Autodesk Fusion 360 part; units mm, degrees
(part 8 of 9)
  spline S13 degree 5 poles (-16.6117, 12.3429) (-16.6198, 12.3478) (-16.6358, 12.3576) (-16.6595, 12.373) (-16.6903, 12.3947) (-16.7276, 12.4235) (-16.7642, 12.4534) (-16.8004, 12.484) (-16.8362, 12.5151) (-16.8719, 12.5464) (-16.9074, 12.578) (-16.9427, 12.61) (-16.9776, 12.6425) (-17.0121, 12.6755) (-17.0463, 12.709) (-17.0801, 12.7431) (-17.1135, 12.7776) (-17.1467, 12.8125) (-17.1796, 12.8477) (-17.2124, 12.8832) (-17.2449, 12.919) (-17.2771, 12.9552) (-17.3091, 12.9916) (-17.3409, 13.0284) (-17.3723, 13.0655) (-17.4036, 13.103) (-17.4346, 13.1407) (-17.4653, 13.1788) (-17.4959, 13.2171) (-17.5262, 13.2557) (-17.5563, 13.2945) (-17.5862, 13.3337) (-17.6158, 13.373) (-17.6453, 13.4127) (-17.6745, 13.4526) (-17.7035, 13.4928) (-17.7323, 13.5332) (-17.7609, 13.5738) (-17.7892, 13.6147) (-17.8174, 13.6559) (-17.8454, 13.6972) (-17.8731, 13.7388) (-17.9007, 13.7807) (-17.928, 13.8227) (-17.9551, 13.865) (-17.9821, 13.9075) (-18.0088, 13.9502) (-18.0354, 13.9931) (-18.0617, 14.0363) (-18.0878, 14.0796) (-18.1138, 14.1232) (-18.1395, 14.1669) (-18.165, 14.2109) (-18.1904, 14.255) (-18.2156, 14.2994) (-18.2405, 14.344) (-18.2653, 14.3887) (-18.2898, 14.4336) (-18.3142, 14.4788) (-18.3384, 14.5241) (-18.3624, 14.5696) (-18.3862, 14.6153) (-18.4098, 14.6612) (-18.4332, 14.7072) (-18.4564, 14.7535) (-18.4795, 14.7999) (-18.5023, 14.8465) (-18.525, 14.8932) (-18.5474, 14.9401) (-18.5697, 14.9873) (-18.5918, 15.0345) (-18.6093, 15.0725) (-18.6224, 15.101) (-18.631, 15.1201) (-18.6354, 15.1296) knots 0 0 0 0 0 0 0.01428571 0.02857143 0.04285714 0.05714286 0.07142857 0.08571429 0.1 0.11428571 0.12857143 0.14285714 0.15714286 0.17142857 0.18571429 0.2 0.21428571 0.22857143 0.24285714 0.25714286 0.27142857 0.28571429 0.3 0.31428571 0.32857143 0.34285714 0.35714286 0.37142857 0.38571429 0.4 0.41428571 0.42857143 0.44285714 0.45714286 0.47142857 0.48571429 0.5 0.51428571 0.52857143 0.54285714 0.55714286 0.57142857 0.58571429 0.6 0.61428571 0.62857143 0.64285714 0.65714286 0.67142857 0.68571429 0.7 0.71428571 0.72857143 0.74285714 0.75714286 0.77142857 0.78571429 0.8 0.81428571 0.82857143 0.84285714 0.85714286 0.87142857 0.88571429 0.9 0.91428571 0.92857143 0.94285714 0.95714286 0.97142857 0.98571429 1 1 1 1 1 1
  line L13 (-16.6117, 12.3429) -> (-16.2962, 12.1549)
  arc A27 (-15.962, 10.9599) -> (-16.2962, 12.1549) centre (-16.757, 11.3818) ccw
  arc A28 (-15.962, 10.9599) -> (-16.228, 10.4378) centre (-0.4607, 2.7328) ccw
  arc A29 (-17.3912, 10.0058) -> (-16.228, 10.4378) centre (-17.0366, 10.833) ccw
  line L14 (-17.3912, 10.0058) -> (-17.7288, 10.1505)
  spline S14 degree 5 poles (-17.7288, 10.1505) (-17.7375, 10.1542) (-17.7549, 10.1614) (-17.7812, 10.1715) (-17.8169, 10.1836) (-17.8621, 10.197) (-17.9078, 10.209) (-17.9538, 10.2202) (-18.0001, 10.231) (-18.0464, 10.2414) (-18.0928, 10.2516) (-18.1394, 10.2613) (-18.1862, 10.2705) (-18.2332, 10.279) (-18.2804, 10.2869) (-18.3278, 10.2942) (-18.3754, 10.301) (-18.4232, 10.3073) (-18.471, 10.3133) (-18.519, 10.3189) (-18.567, 10.3241) (-18.6152, 10.329) (-18.6635, 10.3334) (-18.7119, 10.3375) (-18.7605, 10.3411) (-18.8091, 10.3444) (-18.8579, 10.3473) (-18.9068, 10.3498) (-18.9557, 10.352) (-19.0047, 10.3538) (-19.0539, 10.3553) (-19.1031, 10.3565) (-19.1524, 10.3574) (-19.2018, 10.3579) (-19.2512, 10.3581) (-19.3008, 10.3579) (-19.3504, 10.3575) (-19.4001, 10.3567) (-19.4499, 10.3556) (-19.4997, 10.3542) (-19.5496, 10.3525) (-19.5996, 10.3505) (-19.6496, 10.3482) (-19.6997, 10.3456) (-19.7498, 10.3427) (-19.8, 10.3395) (-19.8503, 10.3361) (-19.9006, 10.3323) (-19.951, 10.3282) (-20.0014, 10.3239) (-20.0519, 10.3193) (-20.1025, 10.3144) (-20.153, 10.3092) (-20.2037, 10.3038) (-20.2543, 10.2981) (-20.3051, 10.2921) (-20.3558, 10.2858) (-20.4066, 10.2793) (-20.4574, 10.2724) (-20.5083, 10.2654) (-20.5592, 10.258) (-20.6102, 10.2504) (-20.6612, 10.2426) (-20.7122, 10.2344) (-20.7633, 10.2261) (-20.8144, 10.2174) (-20.8655, 10.2085) (-20.9166, 10.1994) (-20.9678, 10.1899) (-21.019, 10.1803) (-21.0702, 10.1704) (-21.1112, 10.1622) (-21.142, 10.156) (-21.1625, 10.1518) (-21.1728, 10.1497) knots 0 0 0 0 0 0 0.01428571 0.02857143 0.04285714 0.05714286 0.07142857 0.08571429 0.1 0.11428571 0.12857143 0.14285714 0.15714286 0.17142857 0.18571429 0.2 0.21428571 0.22857143 0.24285714 0.25714286 0.27142857 0.28571429 0.3 0.31428571 0.32857143 0.34285714 0.35714286 0.37142857 0.38571429 0.4 0.41428571 0.42857143 0.44285714 0.45714286 0.47142857 0.48571429 0.5 0.51428571 0.52857143 0.54285714 0.55714286 0.57142857 0.58571429 0.6 0.61428571 0.62857143 0.64285714 0.65714286 0.67142857 0.68571429 0.7 0.71428571 0.72857143 0.74285714 0.75714286 0.77142857 0.78571429 0.8 0.81428571 0.82857143 0.84285714 0.85714286 0.87142857 0.88571429 0.9 0.91428571 0.92857143 0.94285714 0.95714286 0.97142857 0.98571429 1 1 1 1 1 1
  arc A30 (-21.1728, 10.1497) -> (-21.5767, 8.9066) centre (-0.4607, 2.7328) ccw
  spline S15 degree 5 poles (-18.7909, 6.8816) (-18.8001, 6.8837) (-18.8184, 6.8881) (-18.8457, 6.8955) (-18.8816, 6.9066) (-18.9261, 6.9224) (-18.9701, 6.9396) (-19.0139, 6.9575) (-19.0577, 6.976) (-19.1013, 6.9948) (-19.1448, 7.0138) (-19.1882, 7.0334) (-19.2315, 7.0534) (-19.2745, 7.0742) (-19.3174, 7.0955) (-19.36, 7.1175) (-19.4025, 7.14) (-19.4448, 7.1629) (-19.487, 7.1862) (-19.5291, 7.2099) (-19.5711, 7.2339) (-19.6129, 7.2583) (-19.6546, 7.2831) (-19.6962, 7.3082) (-19.7376, 7.3338) (-19.7789, 7.3598) (-19.82, 7.3861) (-19.861, 7.4128) (-19.9019, 7.4398) (-19.9427, 7.4671) (-19.9833, 7.4948) (-20.0238, 7.5228) (-20.0642, 7.551) (-20.1045, 7.5797) (-20.1446, 7.6086) (-20.1846, 7.6378) (-20.2245, 7.6674) (-20.2642, 7.6972) (-20.3038, 7.7273) (-20.3433, 7.7577) (-20.3827, 7.7884) (-20.422, 7.8194) (-20.4611, 7.8507) (-20.5001, 7.8822) (-20.5389, 7.9141) (-20.5777, 7.9462) (-20.6163, 7.9785) (-20.6548, 8.0111) (-20.6932, 8.044) (-20.7315, 8.0772) (-20.7696, 8.1106) (-20.8076, 8.1442) (-20.8455, 8.1782) (-20.8832, 8.2123) (-20.9208, 8.2467) (-20.9584, 8.2814) (-20.9957, 8.3163) (-21.033, 8.3515) (-21.0701, 8.3868) (-21.1071, 8.4225) (-21.144, 8.4583) (-21.1808, 8.4944) (-21.2174, 8.5308) (-21.2539, 8.5673) (-21.2903, 8.6041) (-21.3265, 8.6412) (-21.3626, 8.6784) (-21.3986, 8.7159) (-21.4345, 8.7536) (-21.4702, 8.7915) (-21.5059, 8.8296) (-21.5342, 8.8603) (-21.5555, 8.8834) (-21.5696, 8.8989) (-21.5767, 8.9066) knots 0 0 0 0 0 0 0.01428571 0.02857143 0.04285714 0.05714286 0.07142857 0.08571429 0.1 0.11428571 0.12857143 0.14285714 0.15714286 0.17142857 0.18571429 0.2 0.21428571 0.22857143 0.24285714 0.25714286 0.27142857 0.28571429 0.3 0.31428571 0.32857143 0.34285714 0.35714286 0.37142857 0.38571429 0.4 0.41428571 0.42857143 0.44285714 0.45714286 0.47142857 0.48571429 0.5 0.51428571 0.52857143 0.54285714 0.55714286 0.57142857 0.58571429 0.6 0.61428571 0.62857143 0.64285714 0.65714286 0.67142857 0.68571429 0.7 0.71428571 0.72857143 0.74285714 0.75714286 0.77142857 0.78571429 0.8 0.81428571 0.82857143 0.84285714 0.85714286 0.87142857 0.88571429 0.9 0.91428571 0.92857143 0.94285714 0.95714286 0.97142857 0.98571429 1 1 1 1 1 1
  line L15 (-18.7909, 6.8816) -> (-18.4327, 6.8003)
  arc A31 (-17.7456, 5.767) -> (-18.4327, 6.8003) centre (-18.6321, 5.9227) ccw
  arc A32 (-17.7456, 5.767) -> (-17.8373, 5.1884) centre (-0.4607, 2.7328) ccw
  arc A33 (-18.8101, 4.418) -> (-17.8373, 5.1884) centre (-18.7284, 5.3143) ccw
  line L16 (-18.8101, 4.418) -> (-19.1758, 4.4513)
  spline S16 degree 5 poles (-19.1758, 4.4513) (-19.1852, 4.4522) (-19.204, 4.4536) (-19.2322, 4.4551) (-19.2698, 4.4556) (-19.317, 4.4543) (-19.3642, 4.4516) (-19.4114, 4.4481) (-19.4587, 4.444) (-19.506, 4.4396) (-19.5533, 4.4349) (-19.6006, 4.4298) (-19.6479, 4.4241) (-19.6953, 4.4177) (-19.7426, 4.4106) (-19.79, 4.4029) (-19.8373, 4.3946) (-19.8847, 4.3859) (-19.932, 4.3768) (-19.9794, 4.3673) (-20.0267, 4.3574) (-20.074, 4.3471) (-20.1213, 4.3365) (-20.1686, 4.3253) (-20.2159, 4.3138) (-20.2632, 4.3019) (-20.3105, 4.2895) (-20.3577, 4.2769) (-20.405, 4.2638) (-20.4522, 4.2504) (-20.4994, 4.2367) (-20.5465, 4.2226) (-20.5937, 4.2082) (-20.6408, 4.1934) (-20.6879, 4.1783) (-20.735, 4.1628) (-20.782, 4.1471) (-20.829, 4.131) (-20.876, 4.1145) (-20.923, 4.0978) (-20.9699, 4.0808) (-21.0168, 4.0634) (-21.0637, 4.0458) (-21.1105, 4.0279) (-21.1574, 4.0096) (-21.2041, 3.9911) (-21.2509, 3.9722) (-21.2976, 3.9531) (-21.3442, 3.9337) (-21.3908, 3.914) (-21.4374, 3.894) (-21.484, 3.8737) (-21.5305, 3.8532) (-21.5769, 3.8323) (-21.6234, 3.8112) (-21.6697, 3.7898) (-21.7161, 3.7682) (-21.7624, 3.7463) (-21.8086, 3.7241) (-21.8548, 3.7016) (-21.901, 3.6789) (-21.9471, 3.656) (-21.9932, 3.6327) (-22.0392, 3.6092) (-22.0851, 3.5855) (-22.1311, 3.5615) (-22.1769, 3.5372) (-22.2227, 3.5127) (-22.2685, 3.4879) (-22.3142, 3.4629) (-22.3599, 3.4376) (-22.3963, 3.4172) (-22.4237, 3.4018) (-22.4419, 3.3915) (-22.451, 3.3863) knots 0 0 0 0 0 0 0.01428571 0.02857143 0.04285714 0.05714286 0.07142857 0.08571429 0.1 0.11428571 0.12857143 0.14285714 0.15714286 0.17142857 0.18571429 0.2 0.21428571 0.22857143 0.24285714 0.25714286 0.27142857 0.28571429 0.3 0.31428571 0.32857143 0.34285714 0.35714286 0.37142857 0.38571429 0.4 0.41428571 0.42857143 0.44285714 0.45714286 0.47142857 0.48571429 0.5 0.51428571 0.52857143 0.54285714 0.55714286 0.57142857 0.58571429 0.6 0.61428571 0.62857143 0.64285714 0.65714286 0.67142857 0.68571429 0.7 0.71428571 0.72857143 0.74285714 0.75714286 0.77142857 0.78571429 0.8 0.81428571 0.82857143 0.84285714 0.85714286 0.87142857 0.88571429 0.9 0.91428571 0.92857143 0.94285714 0.95714286 0.97142857 0.98571429 1 1 1 1 1 1
  arc A34 (-22.451, 3.3863) -> (-22.451, 2.0792) centre (-0.4607, 2.7328) ccw
  spline S17 degree 5 poles (-19.1758, 1.0142) (-19.1852, 1.0134) (-19.204, 1.0119) (-19.2322, 1.0105) (-19.2698, 1.01) (-19.317, 1.0112) (-19.3642, 1.0139) (-19.4114, 1.0175) (-19.4587, 1.0215) (-19.506, 1.0259) (-19.5533, 1.0306) (-19.6006, 1.0358) (-19.6479, 1.0415) (-19.6953, 1.0479) (-19.7426, 1.055) (-19.79, 1.0627) (-19.8373, 1.071) (-19.8847, 1.0797) (-19.932, 1.0888) (-19.9794, 1.0983) (-20.0267, 1.1082) (-20.074, 1.1184) (-20.1213, 1.1291) (-20.1686, 1.1402) (-20.2159, 1.1517) (-20.2632, 1.1637) (-20.3105, 1.176) (-20.3577, 1.1887) (-20.405, 1.2018) (-20.4522, 1.2152) (-20.4994, 1.2289) (-20.5465, 1.243) (-20.5937, 1.2574) (-20.6408, 1.2722) (-20.6879, 1.2873) (-20.735, 1.3027) (-20.782, 1.3185) (-20.829, 1.3346) (-20.876, 1.351) (-20.923, 1.3677) (-20.9699, 1.3848) (-21.0168, 1.4021) (-21.0637, 1.4198) (-21.1105, 1.4377) (-21.1574, 1.456) (-21.2041, 1.4745) (-21.2509, 1.4933) (-21.2976, 1.5125) (-21.3442, 1.5319) (-21.3908, 1.5516) (-21.4374, 1.5716) (-21.484, 1.5919) (-21.5305, 1.6124) (-21.5769, 1.6332) (-21.6234, 1.6543) (-21.6697, 1.6757) (-21.7161, 1.6974) (-21.7624, 1.7193) (-21.8086, 1.7415) (-21.8548, 1.7639) (-21.901, 1.7866) (-21.9471, 1.8096) (-21.9932, 1.8328) (-22.0392, 1.8563) (-22.0851, 1.8801) (-22.1311, 1.9041) (-22.1769, 1.9284) (-22.2227, 1.9529) (-22.2685, 1.9776) (-22.3142, 2.0026) (-22.3599, 2.0279) (-22.3963, 2.0483) (-22.4237, 2.0637) (-22.4419, 2.0741) (-22.451, 2.0792) knots 0 0 0 0 0 0 0.01428571 0.02857143 0.04285714 0.05714286 0.07142857 0.08571429 0.1 0.11428571 0.12857143 0.14285714 0.15714286 0.17142857 0.18571429 0.2 0.21428571 0.22857143 0.24285714 0.25714286 0.27142857 0.28571429 0.3 0.31428571 0.32857143 0.34285714 0.35714286 0.37142857 0.38571429 0.4 0.41428571 0.42857143 0.44285714 0.45714286 0.47142857 0.48571429 0.5 0.51428571 0.52857143 0.54285714 0.55714286 0.57142857 0.58571429 0.6 0.61428571 0.62857143 0.64285714 0.65714286 0.67142857 0.68571429 0.7 0.71428571 0.72857143 0.74285714 0.75714286 0.77142857 0.78571429 0.8 0.81428571 0.82857143 0.84285714 0.85714286 0.87142857 0.88571429 0.9 0.91428571 0.92857143 0.94285714 0.95714286 0.97142857 0.98571429 1 1 1 1 1 1
  line L17 (-19.1758, 1.0142) -> (-18.8101, 1.0476)
  arc A35 (-17.8373, 0.2772) -> (-18.8101, 1.0476) centre (-18.7284, 0.1513) ccw
  arc A36 (-17.8373, 0.2772) -> (-17.7456, -0.3015) centre (-0.4607, 2.7328) ccw
  arc A37 (-18.4327, -1.3347) -> (-17.7456, -0.3015) centre (-18.6321, -0.4571) ccw
  line L18 (-18.4327, -1.3347) -> (-18.7909, -1.4161)
  spline S18 degree 5 poles (-18.7909, -1.4161) (-18.8001, -1.4182) (-18.8184, -1.4226) (-18.8457, -1.4299) (-18.8816, -1.4411) (-18.9261, -1.4569) (-18.9701, -1.474) (-19.0139, -1.492) (-19.0577, -1.5104) (-19.1013, -1.5292) (-19.1448, -1.5483) (-19.1882, -1.5678) (-19.2315, -1.5879) (-19.2745, -1.6086) (-19.3174, -1.63) (-19.36, -1.6519) (-19.4025, -1.6744) (-19.4448, -1.6974) (-19.487, -1.7207) (-19.5291, -1.7443) (-19.5711, -1.7683) (-19.6129, -1.7927) (-19.6546, -1.8175) (-19.6962, -1.8427) (-19.7376, -1.8683) (-19.7789, -1.8942) (-19.82, -1.9206) (-19.861, -1.9472) (-19.9019, -1.9742) (-19.9427, -2.0016) (-19.9833, -2.0292) (-20.0238, -2.0572) (-20.0642, -2.0855) (-20.1045, -2.1141) (-20.1446, -2.143) (-20.1846, -2.1723) (-20.2245, -2.2018) (-20.2642, -2.2316) (-20.3038, -2.2618) (-20.3433, -2.2922) (-20.3827, -2.3229) (-20.422, -2.3539) (-20.4611, -2.3851) (-20.5001, -2.4167) (-20.5389, -2.4485) (-20.5777, -2.4806) (-20.6163, -2.513) (-20.6548, -2.5456) (-20.6932, -2.5785) (-20.7315, -2.6116) (-20.7696, -2.645) (-20.8076, -2.6787) (-20.8455, -2.7126) (-20.8832, -2.7468) (-20.9208, -2.7812) (-20.9584, -2.8158) (-20.9957, -2.8507) (-21.033, -2.8859) (-21.0701, -2.9213) (-21.1071, -2.9569) (-21.144, -2.9928) (-21.1808, -3.0289) (-21.2174, -3.0652) (-21.2539, -3.1018) (-21.2903, -3.1386) (-21.3265, -3.1756) (-21.3626, -3.2128) (-21.3986, -3.2503) (-21.4345, -3.288) (-21.4702, -3.3259) (-21.5059, -3.3641) (-21.5342, -3.3947) (-21.5555, -3.4179) (-21.5696, -3.4333) (-21.5767, -3.441) knots 0 0 0 0 0 0 0.01428571 0.02857143 0.04285714 0.05714286 0.07142857 0.08571429 0.1 0.11428571 0.12857143 0.14285714 0.15714286 0.17142857 0.18571429 0.2 0.21428571 0.22857143 0.24285714 0.25714286 0.27142857 0.28571429 0.3 0.31428571 0.32857143 0.34285714 0.35714286 0.37142857 0.38571429 0.4 0.41428571 0.42857143 0.44285714 0.45714286 0.47142857 0.48571429 0.5 0.51428571 0.52857143 0.54285714 0.55714286 0.57142857 0.58571429 0.6 0.61428571 0.62857143 0.64285714 0.65714286 0.67142857 0.68571429 0.7 0.71428571 0.72857143 0.74285714 0.75714286 0.77142857 0.78571429 0.8 0.81428571 0.82857143 0.84285714 0.85714286 0.87142857 0.88571429 0.9 0.91428571 0.92857143 0.94285714 0.95714286 0.97142857 0.98571429 1 1 1 1 1 1
  arc A38 (-21.5767, -3.441) -> (-21.1728, -4.6841) centre (-0.4607, 2.7328) ccw
  spline S19 degree 5 poles (-17.7288, -4.6849) (-17.7375, -4.6886) (-17.7549, -4.6958) (-17.7812, -4.7059) (-17.8169, -4.7181) (-17.8621, -4.7314) (-17.9078, -4.7434) (-17.9538, -4.7546) (-18.0001, -4.7654) (-18.0464, -4.7759) (-18.0928, -4.786) (-18.1394, -4.7957) (-18.1862, -4.8049) (-18.2332, -4.8135) (-18.2804, -4.8213) (-18.3278, -4.8286) (-18.3754, -4.8354) (-18.4232, -4.8417) (-18.471, -4.8477) (-18.519, -4.8533) (-18.567, -4.8585) (-18.6152, -4.8634) (-18.6635, -4.8679) (-18.7119, -4.8719) (-18.7605, -4.8756) (-18.8091, -4.8788) (-18.8579, -4.8817) (-18.9068, -4.8842) (-18.9557, -4.8864) (-19.0047, -4.8883) (-19.0539, -4.8898) (-19.1031, -4.891) (-19.1524, -4.8918) (-19.2018, -4.8923) (-19.2512, -4.8925) (-19.3008, -4.8924) (-19.3504, -4.8919) (-19.4001, -4.8911) (-19.4499, -4.89) (-19.4997, -4.8886) (-19.5496, -4.887) (-19.5996, -4.885) (-19.6496, -4.8827) (-19.6997, -4.8801) (-19.7498, -4.8772) (-19.8, -4.874) (-19.8503, -4.8705) (-19.9006, -4.8667) (-19.951, -4.8627) (-20.0014, -4.8584) (-20.0519, -4.8537) (-20.1025, -4.8488) (-20.153, -4.8437) (-20.2037, -4.8382) (-20.2543, -4.8325) (-20.3051, -4.8265) (-20.3558, -4.8202) (-20.4066, -4.8137) (-20.4574, -4.8069) (-20.5083, -4.7998) (-20.5592, -4.7925) (-20.6102, -4.7849) (-20.6612, -4.777) (-20.7122, -4.7689) (-20.7633, -4.7605) (-20.8144, -4.7519) (-20.8655, -4.743) (-20.9166, -4.7338) (-20.9678, -4.7244) (-21.019, -4.7147) (-21.0702, -4.7048) (-21.1112, -4.6967) (-21.142, -4.6904) (-21.1625, -4.6863) (-21.1728, -4.6841) knots 0 0 0 0 0 0 0.01428571 0.02857143 0.04285714 0.05714286 0.07142857 0.08571429 0.1 0.11428571 0.12857143 0.14285714 0.15714286 0.17142857 0.18571429 0.2 0.21428571 0.22857143 0.24285714 0.25714286 0.27142857 0.28571429 0.3 0.31428571 0.32857143 0.34285714 0.35714286 0.37142857 0.38571429 0.4 0.41428571 0.42857143 0.44285714 0.45714286 0.47142857 0.48571429 0.5 0.51428571 0.52857143 0.54285714 0.55714286 0.57142857 0.58571429 0.6 0.61428571 0.62857143 0.64285714 0.65714286 0.67142857 0.68571429 0.7 0.71428571 0.72857143 0.74285714 0.75714286 0.77142857 0.78571429 0.8 0.81428571 0.82857143 0.84285714 0.85714286 0.87142857 0.88571429 0.9 0.91428571 0.92857143 0.94285714 0.95714286 0.97142857 0.98571429 1 1 1 1 1 1
  line L19 (-17.7288, -4.6849) -> (-17.3912, -4.5402)
  arc A39 (-16.228, -4.9723) -> (-17.3912, -4.5402) centre (-17.0366, -5.3674) ccw
  arc A40 (-16.228, -4.9723) -> (-15.962, -5.4943) centre (-0.4607, 2.7328) ccw
  arc A41 (-16.2962, -6.6893) -> (-15.962, -5.4943) centre (-16.757, -5.9162) ccw
  line L20 (-16.2962, -6.6893) -> (-16.6117, -6.8774)
  spline S20 degree 5 poles (-16.6117, -6.8774) (-16.6198, -6.8822) (-16.6358, -6.892) (-16.6595, -6.9074) (-16.6903, -6.9292) (-16.7276, -6.9579) (-16.7642, -6.9878) (-16.8004, -7.0185) (-16.8362, -7.0495) (-16.8719, -7.0809) (-16.9074, -7.1125) (-16.9427, -7.1444) (-16.9776, -7.1769) (-17.0121, -7.2099) (-17.0463, -7.2435) (-17.0801, -7.2775) (-17.1135, -7.3121) (-17.1467, -7.3469) (-17.1796, -7.3822) (-17.2124, -7.4177) (-17.2449, -7.4535) (-17.2771, -7.4896) (-17.3091, -7.526) (-17.3409, -7.5628) (-17.3723, -7.6) (-17.4036, -7.6374) (-17.4346, -7.6752) (-17.4653, -7.7132) (-17.4959, -7.7515) (-17.5262, -7.7901) (-17.5563, -7.829) (-17.5862, -7.8681) (-17.6158, -7.9075) (-17.6453, -7.9471) (-17.6745, -7.987) (-17.7035, -8.0272) (-17.7323, -8.0676) (-17.7609, -8.1083) (-17.7892, -8.1492) (-17.8174, -8.1903) (-17.8454, -8.2317) (-17.8731, -8.2733) (-17.9007, -8.3151) (-17.928, -8.3572) (-17.9551, -8.3994) (-17.9821, -8.4419) (-18.0088, -8.4846) (-18.0354, -8.5276) (-18.0617, -8.5707) (-18.0878, -8.614) (-18.1138, -8.6576) (-18.1395, -8.7014) (-18.165, -8.7453) (-18.1904, -8.7895) (-18.2156, -8.8338) (-18.2405, -8.8784) (-18.2653, -8.9231) (-18.2898, -8.9681) (-18.3142, -9.0132) (-18.3384, -9.0585) (-18.3624, -9.104) (-18.3862, -9.1497) (-18.4098, -9.1956) (-18.4332, -9.2417) (-18.4564, -9.2879) (-18.4795, -9.3343) (-18.5023, -9.3809) (-18.525, -9.4277) (-18.5474, -9.4746) (-18.5697, -9.5217) (-18.5918, -9.569) (-18.6093, -9.6069) (-18.6224, -9.6355) (-18.631, -9.6545) (-18.6354, -9.6641) knots 0 0 0 0 0 0 0.01428571 0.02857143 0.04285714 0.05714286 0.07142857 0.08571429 0.1 0.11428571 0.12857143 0.14285714 0.15714286 0.17142857 0.18571429 0.2 0.21428571 0.22857143 0.24285714 0.25714286 0.27142857 0.28571429 0.3 0.31428571 0.32857143 0.34285714 0.35714286 0.37142857 0.38571429 0.4 0.41428571 0.42857143 0.44285714 0.45714286 0.47142857 0.48571429 0.5 0.51428571 0.52857143 0.54285714 0.55714286 0.57142857 0.58571429 0.6 0.61428571 0.62857143 0.64285714 0.65714286 0.67142857 0.68571429 0.7 0.71428571 0.72857143 0.74285714 0.75714286 0.77142857 0.78571429 0.8 0.81428571 0.82857143 0.84285714 0.85714286 0.87142857 0.88571429 0.9 0.91428571 0.92857143 0.94285714 0.95714286 0.97142857 0.98571429 1 1 1 1 1 1
  arc A42 (-18.6354, -9.6641) -> (-17.8671, -10.7215) centre (-0.4607, 2.7328) ccw
  spline S21 degree 5 poles (-14.5914, -9.658) (-14.5985, -9.6642) (-14.6129, -9.6764) (-14.6348, -9.6942) (-14.665, -9.7167) (-14.7039, -9.7434) (-14.7436, -9.769) (-14.7839, -9.7938) (-14.8246, -9.8184) (-14.8654, -9.8426) (-14.9064, -9.8666) (-14.9477, -9.8903) (-14.9894, -9.9135) (-15.0314, -9.9361) (-15.0739, -9.9582) (-15.1168, -9.9798) (-15.1599, -10.0009) (-15.2034, -10.0217) (-15.247, -10.0422) (-15.2909, -10.0623) (-15.335, -10.0822) (-15.3793, -10.1017) (-15.4239, -10.1208) (-15.4687, -10.1397) (-15.5137, -10.1581) (-15.559, -10.1763) (-15.6045, -10.1941) (-15.6502, -10.2116) (-15.696, -10.2288) (-15.7421, -10.2457) (-15.7884, -10.2623) (-15.8348, -10.2786) (-15.8814, -10.2947) (-15.9282, -10.3104) (-15.9752, -10.3259) (-16.0224, -10.3411) (-16.0697, -10.356) (-16.1172, -10.3706) (-16.1649, -10.3849) (-16.2127, -10.399) (-16.2607, -10.4128) (-16.3088, -10.4263) (-16.3571, -10.4396) (-16.4056, -10.4526) (-16.4541, -10.4654) (-16.5029, -10.4779) (-16.5518, -10.4901) (-16.6008, -10.5021) (-16.65, -10.5138) (-16.6993, -10.5252) (-16.7487, -10.5364) (-16.7983, -10.5474) (-16.848, -10.5581) (-16.8978, -10.5686) (-16.9478, -10.5788) (-16.9979, -10.5888) (-17.0481, -10.5985) (-17.0984, -10.608) (-17.1489, -10.6172) (-17.1994, -10.6262) (-17.2501, -10.635) (-17.3009, -10.6435) (-17.3519, -10.6517) (-17.4029, -10.6598) (-17.454, -10.6676) (-17.5053, -10.6752) (-17.5567, -10.6825) (-17.6081, -10.6896) (-17.6597, -10.6964) (-17.7114, -10.7031) (-17.7632, -10.7095) (-17.8047, -10.7144) (-17.8359, -10.718) (-17.8567, -10.7203) (-17.8671, -10.7215) knots 0 0 0 0 0 0 0.01428571 0.02857143 0.04285714 0.05714286 0.07142857 0.08571429 0.1 0.11428571 0.12857143 0.14285714 0.15714286 0.17142857 0.18571429 0.2 0.21428571 0.22857143 0.24285714 0.25714286 0.27142857 0.28571429 0.3 0.31428571 0.32857143 0.34285714 0.35714286 0.37142857 0.38571429 0.4 0.41428571 0.42857143 0.44285714 0.45714286 0.47142857 0.48571429 0.5 0.51428571 0.52857143 0.54285714 0.55714286 0.57142857 0.58571429 0.6 0.61428571 0.62857143 0.64285714 0.65714286 0.67142857 0.68571429 0.7 0.71428571 0.72857143 0.74285714 0.75714286 0.77142857 0.78571429 0.8 0.81428571 0.82857143 0.84285714 0.85714286 0.87142857 0.88571429 0.9 0.91428571 0.92857143 0.94285714 0.95714286 0.97142857 0.98571429 1 1 1 1 1 1
  line L21 (-14.5914, -9.658) -> (-14.3151, -9.4161)
  arc A43 (-13.0753, -9.4675) -> (-14.3151, -9.4161) centre (-13.7222, -10.0932) ccw
  arc A44 (-13.0753, -9.4675) -> (-12.661, -9.8818) centre (-0.4607, 2.7328) ccw
  arc A45 (-12.6096, -11.1216) -> (-12.661, -9.8818) centre (-13.2867, -10.5287) ccw
  line L22 (-12.6096, -11.1216) -> (-12.8515, -11.3979)
  spline S22 degree 5 poles (-12.8515, -11.3979) (-12.8577, -11.405) (-12.8699, -11.4194) (-12.8877, -11.4413) (-12.9102, -11.4715) (-12.9369, -11.5104) (-12.9625, -11.5501) (-12.9873, -11.5904) (-13.0119, -11.6311) (-13.0361, -11.6719) (-13.0601, -11.7129) (-13.0838, -11.7542) (-13.107, -11.7959) (-13.1296, -11.8379) (-13.1517, -11.8804) (-13.1733, -11.9233) (-13.1944, -11.9664) (-13.2152, -12.0099) (-13.2357, -12.0535) (-13.2558, -12.0974) (-13.2757, -12.1415) (-13.2952, -12.1858) (-13.3143, -12.2304) (-13.3332, -12.2752) (-13.3516, -12.3202) (-13.3698, -12.3655) (-13.3876, -12.411) (-13.4051, -12.4567) (-13.4223, -12.5025) (-13.4392, -12.5486) (-13.4558, -12.5949) (-13.4721, -12.6413) (-13.4882, -12.6879) (-13.5039, -12.7347) (-13.5194, -12.7817) (-13.5346, -12.8289) (-13.5495, -12.8762) (-13.5641, -12.9237) (-13.5784, -12.9714) (-13.5925, -13.0192) (-13.6063, -13.0672) (-13.6198, -13.1153) (-13.6331, -13.1636) (-13.6461, -13.2121) (-13.6589, -13.2607) (-13.6714, -13.3094) (-13.6836, -13.3583) (-13.6956, -13.4073) (-13.7073, -13.4565) (-13.7187, -13.5058) (-13.7299, -13.5552) (-13.7409, -13.6048) (-13.7516, -13.6545) (-13.7621, -13.7043) (-13.7723, -13.7543) (-13.7823, -13.8044) (-13.792, -13.8546) (-13.8015, -13.9049) (-13.8107, -13.9554) (-13.8197, -14.0059) (-13.8284, -14.0566) (-13.837, -14.1074) (-13.8452, -14.1584) (-13.8533, -14.2094) (-13.8611, -14.2605) (-13.8686, -14.3118) (-13.876, -14.3632) (-13.8831, -14.4146) (-13.8899, -14.4662) (-13.8966, -14.5179) (-13.903, -14.5697) (-13.9079, -14.6112) (-13.9115, -14.6424) (-13.9138, -14.6632) (-13.915, -14.6736) knots 0 0 0 0 0 0 0.01428571 0.02857143 0.04285714 0.05714286 0.07142857 0.08571429 0.1 0.11428571 0.12857143 0.14285714 0.15714286 0.17142857 0.18571429 0.2 0.21428571 0.22857143 0.24285714 0.25714286 0.27142857 0.28571429 0.3 0.31428571 0.32857143 0.34285714 0.35714286 0.37142857 0.38571429 0.4 0.41428571 0.42857143 0.44285714 0.45714286 0.47142857 0.48571429 0.5 0.51428571 0.52857143 0.54285714 0.55714286 0.57142857 0.58571429 0.6 0.61428571 0.62857143 0.64285714 0.65714286 0.67142857 0.68571429 0.7 0.71428571 0.72857143 0.74285714 0.75714286 0.77142857 0.78571429 0.8 0.81428571 0.82857143 0.84285714 0.85714286 0.87142857 0.88571429 0.9 0.91428571 0.92857143 0.94285714 0.95714286 0.97142857 0.98571429 1 1 1 1 1 1
  arc A46 (-13.915, -14.6736) -> (-12.8576, -15.4419) centre (-0.4607, 2.7328) ccw
  spline S23 degree 5 poles (-10.0709, -13.4182) (-10.0757, -13.4263) (-10.0855, -13.4423) (-10.1009, -13.466) (-10.1227, -13.4968) (-10.1514, -13.5341) (-10.1813, -13.5707) (-10.212, -13.6069) (-10.243, -13.6427) (-10.2743, -13.6784) (-10.306, -13.7139) (-10.3379, -13.7492) (-10.3704, -13.7841) (-10.4034, -13.8187) (-10.437, -13.8528) (-10.471, -13.8866) (-10.5056, -13.92) (-10.5404, -13.9532) (-10.5757, -13.9861) (-10.6112, -14.0189) (-10.647, -14.0514) (-10.6831, -14.0836) (-10.7195, -14.1156) (-10.7563, -14.1474) (-10.7935, -14.1788) (-10.8309, -14.2101) (-10.8687, -14.2411) (-10.9067, -14.2718) (-10.945, -14.3024) (-10.9836, -14.3327) (-11.0225, -14.3628) (-11.0616, -14.3927) (-11.101, -14.4223) (-11.1406, -14.4518) (-11.1805, -14.481) (-11.2207, -14.51) (-11.2611, -14.5388) (-11.3018, -14.5674) (-11.3427, -14.5958) (-11.3838, -14.6239) (-11.4252, -14.6519) (-11.4668, -14.6796) (-11.5086, -14.7072) (-11.5506, -14.7345) (-11.5929, -14.7617) (-11.6354, -14.7886) (-11.6781, -14.8153) (-11.7211, -14.8419) (-11.7642, -14.8682) (-11.8075, -14.8943) (-11.8511, -14.9203) (-11.8948, -14.946) (-11.9388, -14.9716) (-11.983, -14.9969) (-12.0273, -15.0221) (-12.0719, -15.047) (-12.1166, -15.0718) (-12.1616, -15.0963) (-12.2067, -15.1207) (-12.252, -15.1449) (-12.2975, -15.1689) (-12.3432, -15.1927) (-12.3891, -15.2163) (-12.4352, -15.2397) (-12.4814, -15.263) (-12.5278, -15.286) (-12.5744, -15.3088) (-12.6211, -15.3315) (-12.6681, -15.354) (-12.7152, -15.3762) (-12.7625, -15.3983) (-12.8004, -15.4158) (-12.829, -15.4289) (-12.848, -15.4376) (-12.8576, -15.4419) knots 0 0 0 0 0 0 0.01428571 0.02857143 0.04285714 0.05714286 0.07142857 0.08571429 0.1 0.11428571 0.12857143 0.14285714 0.15714286 0.17142857 0.18571429 0.2 0.21428571 0.22857143 0.24285714 0.25714286 0.27142857 0.28571429 0.3 0.31428571 0.32857143 0.34285714 0.35714286 0.37142857 0.38571429 0.4 0.41428571 0.42857143 0.44285714 0.45714286 0.47142857 0.48571429 0.5 0.51428571 0.52857143 0.54285714 0.55714286 0.57142857 0.58571429 0.6 0.61428571 0.62857143 0.64285714 0.65714286 0.67142857 0.68571429 0.7 0.71428571 0.72857143 0.74285714 0.75714286 0.77142857 0.78571429 0.8 0.81428571 0.82857143 0.84285714 0.85714286 0.87142857 0.88571429 0.9 0.91428571 0.92857143 0.94285714 0.95714286 0.97142857 0.98571429 1 1 1 1 1 1
  line L23 (-10.0709, -13.4182) -> (-9.8828, -13.1027)
  arc A47 (-8.6878, -12.7685) -> (-9.8828, -13.1027) centre (-9.1097, -13.5635) ccw
  arc A48 (-8.6878, -12.7685) -> (-8.1657, -13.0345) centre (-0.4607, 2.7328) ccw
  arc A49 (-7.7337, -14.1977) -> (-8.1657, -13.0345) centre (-8.5609, -13.8431) ccw
  line L24 (-7.7337, -14.1977) -> (-7.8784, -14.5353)
  spline S24 degree 5 poles (-7.8784, -14.5353) (-7.8821, -14.544) (-7.8893, -14.5614) (-7.8994, -14.5877) (-7.9116, -14.6234) (-7.9249, -14.6686) (-7.9369, -14.7143) (-7.9481, -14.7604) (-7.9589, -14.8066) (-7.9693, -14.8529) (-7.9795, -14.8993) (-7.9892, -14.9459) (-7.9984, -14.9927) (-8.0069, -15.0397) (-8.0148, -15.0869) (-8.0221, -15.1343) (-8.0289, -15.1819) (-8.0352, -15.2297) (-8.0412, -15.2775) (-8.0468, -15.3255) (-8.052, -15.3735) (-8.0569, -15.4217) (-8.0614, -15.47) (-8.0654, -15.5184) (-8.0691, -15.567) (-8.0723, -15.6156) (-8.0752, -15.6644) (-8.0777, -15.7133) (-8.0799, -15.7622) (-8.0818, -15.8113) (-8.0833, -15.8604) (-8.0845, -15.9096) (-8.0853, -15.9589) (-8.0858, -16.0083) (-8.086, -16.0577) (-8.0859, -16.1073) (-8.0854, -16.1569) (-8.0846, -16.2066) (-8.0835, -16.2564) (-8.0821, -16.3062) (-8.0804, -16.3561) (-8.0784, -16.4061) (-8.0761, -16.4561) (-8.0736, -16.5062) (-8.0707, -16.5563) (-8.0675, -16.6065) (-8.064, -16.6568) (-8.0602, -16.7071) (-8.0562, -16.7575) (-8.0518, -16.8079) (-8.0472, -16.8584) (-8.0423, -16.909) (-8.0372, -16.9595) (-8.0317, -17.0102) (-8.026, -17.0608) (-8.02, -17.1116) (-8.0137, -17.1623) (-8.0072, -17.2131) (-8.0004, -17.264) (-7.9933, -17.3148) (-7.986, -17.3658) (-7.9784, -17.4167) (-7.9705, -17.4677) (-7.9624, -17.5187) (-7.954, -17.5698) (-7.9453, -17.6209) (-7.9364, -17.672) (-7.9273, -17.7231) (-7.9179, -17.7743) (-7.9082, -17.8255) (-7.8983, -17.8767) (-7.8902, -17.9177) (-7.8839, -17.9485) (-7.8797, -17.969) (-7.8776, -17.9793) knots 0 0 0 0 0 0 0.01428571 0.02857143 0.04285714 0.05714286 0.07142857 0.08571429 0.1 0.11428571 0.12857143 0.14285714 0.15714286 0.17142857 0.18571429 0.2 0.21428571 0.22857143 0.24285714 0.25714286 0.27142857 0.28571429 0.3 0.31428571 0.32857143 0.34285714 0.35714286 0.37142857 0.38571429 0.4 0.41428571 0.42857143 0.44285714 0.45714286 0.47142857 0.48571429 0.5 0.51428571 0.52857143 0.54285714 0.55714286 0.57142857 0.58571429 0.6 0.61428571 0.62857143 0.64285714 0.65714286 0.67142857 0.68571429 0.7 0.71428571 0.72857143 0.74285714 0.75714286 0.77142857 0.78571429 0.8 0.81428571 0.82857143 0.84285714 0.85714286 0.87142857 0.88571429 0.9 0.91428571 0.92857143 0.94285714 0.95714286 0.97142857 0.98571429 1 1 1 1 1 1
  arc A50 (-7.8776, -17.9793) -> (-6.6345, -18.3832) centre (-0.4607, 2.7328) ccw
  spline S25 degree 5 poles (-4.6096, -15.5974) (-4.6117, -15.6066) (-4.6161, -15.6249) (-4.6234, -15.6522) (-4.6346, -15.6881) (-4.6503, -15.7326) (-4.6675, -15.7766) (-4.6855, -15.8205) (-4.7039, -15.8642) (-4.7227, -15.9078) (-4.7418, -15.9513) (-4.7613, -15.9947) (-4.7814, -16.038) (-4.8021, -16.081) (-4.8235, -16.1239) (-4.8454, -16.1665) (-4.8679, -16.209) (-4.8909, -16.2513) (-4.9142, -16.2936) (-4.9378, -16.3356) (-4.9618, -16.3776) (-4.9862, -16.4194) (-5.011, -16.4612) (-5.0362, -16.5027) (-5.0618, -16.5441) (-5.0877, -16.5854) (-5.1141, -16.6265) (-5.1407, -16.6676) (-5.1677, -16.7084) (-5.1951, -16.7492) (-5.2227, -16.7898) (-5.2507, -16.8303) (-5.279, -16.8707) (-5.3076, -16.911) (-5.3365, -16.9511) (-5.3658, -16.9911) (-5.3953, -17.031) (-5.4251, -17.0707) (-5.4553, -17.1103) (-5.4857, -17.1498) (-5.5164, -17.1892) (-5.5474, -17.2285) (-5.5786, -17.2676) (-5.6102, -17.3066) (-5.642, -17.3455) (-5.6741, -17.3842) (-5.7064, -17.4228) (-5.7391, -17.4613) (-5.772, -17.4997) (-5.8051, -17.538) (-5.8385, -17.5761) (-5.8722, -17.6141) (-5.9061, -17.652) (-5.9403, -17.6897) (-5.9747, -17.7274) (-6.0093, -17.7649) (-6.0442, -17.8022) (-6.0794, -17.8395) (-6.1148, -17.8766) (-6.1504, -17.9136) (-6.1863, -17.9505) (-6.2224, -17.9873) (-6.2587, -18.0239) (-6.2953, -18.0604) (-6.3321, -18.0968) (-6.3691, -18.133) (-6.4063, -18.1691) (-6.4438, -18.2051) (-6.4815, -18.241) (-6.5194, -18.2767) (-6.5576, -18.3124) (-6.5882, -18.3408) (-6.6113, -18.362) (-6.6268, -18.3761) (-6.6345, -18.3832) knots 0 0 0 0 0 0 0.01428571 0.02857143 0.04285714 0.05714286 0.07142857 0.08571429 0.1 0.11428571 0.12857143 0.14285714 0.15714286 0.17142857 0.18571429 0.2 0.21428571 0.22857143 0.24285714 0.25714286 0.27142857 0.28571429 0.3 0.31428571 0.32857143 0.34285714 0.35714286 0.37142857 0.38571429 0.4 0.41428571 0.42857143 0.44285714 0.45714286 0.47142857 0.48571429 0.5 0.51428571 0.52857143 0.54285714 0.55714286 0.57142857 0.58571429 0.6 0.61428571 0.62857143 0.64285714 0.65714286 0.67142857 0.68571429 0.7 0.71428571 0.72857143 0.74285714 0.75714286 0.77142857 0.78571429 0.8 0.81428571 0.82857143 0.84285714 0.85714286 0.87142857 0.88571429 0.9 0.91428571 0.92857143 0.94285714 0.95714286 0.97142857 0.98571429 1 1 1 1 1 1
  line L25 (-4.6096, -15.5974) -> (-4.5282, -15.2392)
  arc A51 (-3.495, -14.5521) -> (-4.5282, -15.2392) centre (-3.6506, -15.4386) ccw
  arc A52 (-3.495, -14.5521) -> (-2.9163, -14.6438) centre (-0.4607, 2.7328) ccw
  arc A53 (-2.1459, -15.6166) -> (-2.9163, -14.6438) centre (-3.0422, -15.5349) ccw
  line L26 (-2.1459, -15.6166) -> (-2.1792, -15.9823)
  spline S26 degree 5 poles (-2.1792, -15.9823) (-2.1801, -15.9917) (-2.1816, -16.0105) (-2.183, -16.0387) (-2.1835, -16.0763) (-2.1822, -16.1235) (-2.1796, -16.1707) (-2.176, -16.2179) (-2.1719, -16.2652) (-2.1676, -16.3125) (-2.1629, -16.3598) (-2.1577, -16.4071) (-2.152, -16.4544) (-2.1456, -16.5018) (-2.1385, -16.5491) (-2.1308, -16.5965) (-2.1225, -16.6438) (-2.1138, -16.6912) (-2.1047, -16.7385) (-2.0952, -16.7859) (-2.0853, -16.8332) (-2.0751, -16.8805) (-2.0644, -16.9278) (-2.0533, -16.9752) (-2.0417, -17.0224) (-2.0298, -17.0697) (-2.0175, -17.117) (-2.0048, -17.1642) (-1.9917, -17.2115) (-1.9783, -17.2587) (-1.9646, -17.3059) (-1.9505, -17.353) (-1.9361, -17.4002) (-1.9213, -17.4473) (-1.9062, -17.4944) (-1.8908, -17.5415) (-1.875, -17.5885) (-1.8589, -17.6356) (-1.8425, -17.6825) (-1.8258, -17.7295) (-1.8087, -17.7764) (-1.7914, -17.8233) (-1.7737, -17.8702) (-1.7558, -17.9171) (-1.7375, -17.9639) (-1.719, -18.0106) (-1.7002, -18.0574) (-1.681, -18.1041) (-1.6616, -18.1507) (-1.6419, -18.1973) (-1.6219, -18.2439) (-1.6016, -18.2905) (-1.5811, -18.337) (-1.5603, -18.3834) (-1.5392, -18.4299) (-1.5178, -18.4763) (-1.4961, -18.5226) (-1.4742, -18.5689) (-1.452, -18.6151) (-1.4296, -18.6613) (-1.4069, -18.7075) (-1.3839, -18.7536) (-1.3607, -18.7997) (-1.3372, -18.8457) (-1.3134, -18.8916) (-1.2894, -18.9376) (-1.2651, -18.9834) (-1.2406, -19.0292) (-1.2159, -19.075) (-1.1908, -19.1207) (-1.1656, -19.1664) (-1.1452, -19.2029) (-1.1298, -19.2302) (-1.1194, -19.2484) (-1.1142, -19.2575) knots 0 0 0 0 0 0 0.01428571 0.02857143 0.04285714 0.05714286 0.07142857 0.08571429 0.1 0.11428571 0.12857143 0.14285714 0.15714286 0.17142857 0.18571429 0.2 0.21428571 0.22857143 0.24285714 0.25714286 0.27142857 0.28571429 0.3 0.31428571 0.32857143 0.34285714 0.35714286 0.37142857 0.38571429 0.4 0.41428571 0.42857143 0.44285714 0.45714286 0.47142857 0.48571429 0.5 0.51428571 0.52857143 0.54285714 0.55714286 0.57142857 0.58571429 0.6 0.61428571 0.62857143 0.64285714 0.65714286 0.67142857 0.68571429 0.7 0.71428571 0.72857143 0.74285714 0.75714286 0.77142857 0.78571429 0.8 0.81428571 0.82857143 0.84285714 0.85714286 0.87142857 0.88571429 0.9 0.91428571 0.92857143 0.94285714 0.95714286 0.97142857 0.98571429 1 1 1 1 1 1
  arc A54 (-1.1142, -19.2575) -> (0.1928, -19.2575) centre (-0.4607, 2.7328) ccw
  spline S27 degree 5 poles (1.2578, -15.9823) (1.2587, -15.9917) (1.2601, -16.0105) (1.2616, -16.0387) (1.2621, -16.0763) (1.2608, -16.1235) (1.2581, -16.1707) (1.2546, -16.2179) (1.2505, -16.2652) (1.2462, -16.3125) (1.2415, -16.3598) (1.2363, -16.4071) (1.2306, -16.4544) (1.2242, -16.5018) (1.2171, -16.5491) (1.2094, -16.5965) (1.2011, -16.6438) (1.1924, -16.6912) (1.1833, -16.7385) (1.1738, -16.7859) (1.1639, -16.8332) (1.1536, -16.8805) (1.143, -16.9278) (1.1319, -16.9752) (1.1203, -17.0224) (1.1084, -17.0697) (1.0961, -17.117) (1.0834, -17.1642) (1.0703, -17.2115) (1.0569, -17.2587) (1.0432, -17.3059) (1.0291, -17.353) (1.0147, -17.4002) (0.9999, -17.4473) (0.9848, -17.4944) (0.9693, -17.5415) (0.9536, -17.5885) (0.9375, -17.6356) (0.9211, -17.6825) (0.9043, -17.7295) (0.8873, -17.7764) (0.87, -17.8233) (0.8523, -17.8702) (0.8344, -17.9171) (0.8161, -17.9639) (0.7976, -18.0106) (0.7787, -18.0574) (0.7596, -18.1041) (0.7402, -18.1507) (0.7205, -18.1973) (0.7005, -18.2439) (0.6802, -18.2905) (0.6597, -18.337) (0.6388, -18.3834) (0.6177, -18.4299) (0.5964, -18.4763) (0.5747, -18.5226) (0.5528, -18.5689) (0.5306, -18.6151) (0.5082, -18.6613) (0.4854, -18.7075) (0.4625, -18.7536) (0.4392, -18.7997) (0.4157, -18.8457) (0.392, -18.8916) (0.368, -18.9376) (0.3437, -18.9834) (0.3192, -19.0292) (0.2944, -19.075) (0.2694, -19.1207) (0.2442, -19.1664) (0.2237, -19.2029) (0.2083, -19.2302) (0.198, -19.2484) (0.1928, -19.2575) knots 0 0 0 0 0 0 0.01428571 0.02857143 0.04285714 0.05714286 0.07142857 0.08571429 0.1 0.11428571 0.12857143 0.14285714 0.15714286 0.17142857 0.18571429 0.2 0.21428571 0.22857143 0.24285714 0.25714286 0.27142857 0.28571429 0.3 0.31428571 0.32857143 0.34285714 0.35714286 0.37142857 0.38571429 0.4 0.41428571 0.42857143 0.44285714 0.45714286 0.47142857 0.48571429 0.5 0.51428571 0.52857143 0.54285714 0.55714286 0.57142857 0.58571429 0.6 0.61428571 0.62857143 0.64285714 0.65714286 0.67142857 0.68571429 0.7 0.71428571 0.72857143 0.74285714 0.75714286 0.77142857 0.78571429 0.8 0.81428571 0.82857143 0.84285714 0.85714286 0.87142857 0.88571429 0.9 0.91428571 0.92857143 0.94285714 0.95714286 0.97142857 0.98571429 1 1 1 1 1 1
  line L27 (1.2578, -15.9823) -> (1.2245, -15.6166)
  arc A55 (1.9949, -14.6438) -> (1.2245, -15.6166) centre (2.1208, -15.5349) ccw
  arc A56 (1.9949, -14.6438) -> (2.5736, -14.5521) centre (-0.4607, 2.7328) ccw
  arc A57 (3.6068, -15.2392) -> (2.5736, -14.5521) centre (2.7292, -15.4386) ccw
  line L28 (3.6068, -15.2392) -> (3.6882, -15.5974)
  spline S28 degree 5 poles (3.6882, -15.5974) (3.6902, -15.6066) (3.6947, -15.6249) (3.702, -15.6522) (3.7131, -15.6881) (3.7289, -15.7326) (3.7461, -15.7766) (3.764, -15.8205) (3.7825, -15.8642) (3.8013, -15.9078) (3.8204, -15.9513) (3.8399, -15.9947) (3.8599, -16.038) (3.8807, -16.081) (3.902, -16.1239) (3.924, -16.1665) (3.9465, -16.209) (3.9694, -16.2513) (3.9927, -16.2936) (4.0164, -16.3356) (4.0404, -16.3776) (4.0648, -16.4194) (4.0896, -16.4612) (4.1148, -16.5027) (4.1403, -16.5441) (4.1663, -16.5854) (4.1926, -16.6265) (4.2193, -16.6676) (4.2463, -16.7084) (4.2736, -16.7492) (4.3013, -16.7898) (4.3293, -16.8303) (4.3576, -16.8707) (4.3862, -16.911) (4.4151, -16.9511) (4.4443, -16.9911) (4.4739, -17.031) (4.5037, -17.0707) (4.5338, -17.1103) (4.5642, -17.1498) (4.595, -17.1892) (4.6259, -17.2285) (4.6572, -17.2676) (4.6887, -17.3066) (4.7206, -17.3455) (4.7527, -17.3842) (4.785, -17.4228) (4.8176, -17.4613) (4.8505, -17.4997) (4.8837, -17.538) (4.9171, -17.5761) (4.9508, -17.6141) (4.9847, -17.652) (5.0188, -17.6897) (5.0532, -17.7274) (5.0879, -17.7649) (5.1228, -17.8022) (5.158, -17.8395) (5.1934, -17.8766) (5.229, -17.9136) (5.2648, -17.9505) (5.3009, -17.9873) (5.3373, -18.0239) (5.3738, -18.0604) (5.4106, -18.0968) (5.4477, -18.133) (5.4849, -18.1691) (5.5224, -18.2051) (5.5601, -18.241) (5.598, -18.2767) (5.6361, -18.3124) (5.6668, -18.3408) (5.6899, -18.362) (5.7054, -18.3761) (5.7131, -18.3832) knots 0 0 0 0 0 0 0.01428571 0.02857143 0.04285714 0.05714286 0.07142857 0.08571429 0.1 0.11428571 0.12857143 0.14285714 0.15714286 0.17142857 0.18571429 0.2 0.21428571 0.22857143 0.24285714 0.25714286 0.27142857 0.28571429 0.3 0.31428571 0.32857143 0.34285714 0.35714286 0.37142857 0.38571429 0.4 0.41428571 0.42857143 0.44285714 0.45714286 0.47142857 0.48571429 0.5 0.51428571 0.52857143 0.54285714 0.55714286 0.57142857 0.58571429 0.6 0.61428571 0.62857143 0.64285714 0.65714286 0.67142857 0.68571429 0.7 0.71428571 0.72857143 0.74285714 0.75714286 0.77142857 0.78571429 0.8 0.81428571 0.82857143 0.84285714 0.85714286 0.87142857 0.88571429 0.9 0.91428571 0.92857143 0.94285714 0.95714286 0.97142857 0.98571429 1 1 1 1 1 1
  arc A58 (5.7131, -18.3832) -> (6.9562, -17.9793) centre (-0.4607, 2.7328) ccw
  spline S29 degree 5 poles (6.957, -14.5353) (6.9607, -14.544) (6.9679, -14.5614) (6.978, -14.5877) (6.9901, -14.6234) (7.0035, -14.6686) (7.0155, -14.7143) (7.0267, -14.7604) (7.0375, -14.8066) (7.0479, -14.8529) (7.0581, -14.8993) (7.0678, -14.9459) (7.077, -14.9927) (7.0855, -15.0397) (7.0934, -15.0869) (7.1007, -15.1343) (7.1075, -15.1819) (7.1138, -15.2297) (7.1198, -15.2775) (7.1254, -15.3255) (7.1306, -15.3735) (7.1355, -15.4217) (7.1399, -15.47) (7.144, -15.5184) (7.1476, -15.567) (7.1509, -15.6156) (7.1538, -15.6644) (7.1563, -15.7133) (7.1585, -15.7622) (7.1603, -15.8113) (7.1619, -15.8604) (7.163, -15.9096) (7.1639, -15.9589) (7.1644, -16.0083) (7.1646, -16.0577) (7.1644, -16.1073) (7.164, -16.1569) (7.1632, -16.2066) (7.1621, -16.2564) (7.1607, -16.3062) (7.159, -16.3561) (7.157, -16.4061) (7.1547, -16.4561) (7.1521, -16.5062) (7.1492, -16.5563) (7.146, -16.6065) (7.1426, -16.6568) (7.1388, -16.7071) (7.1348, -16.7575) (7.1304, -16.8079) (7.1258, -16.8584) (7.1209, -16.909) (7.1157, -16.9595) (7.1103, -17.0102) (7.1046, -17.0608) (7.0986, -17.1116) (7.0923, -17.1623) (7.0858, -17.2131) (7.079, -17.264) (7.0719, -17.3148) (7.0645, -17.3658) (7.0569, -17.4167) (7.0491, -17.4677) (7.041, -17.5187) (7.0326, -17.5698) (7.0239, -17.6209) (7.015, -17.672) (7.0059, -17.7231) (6.9964, -17.7743) (6.9868, -17.8255) (6.9769, -17.8767) (6.9687, -17.9177) (6.9625, -17.9485) (6.9583, -17.969) (6.9562, -17.9793) knots 0 0 0 0 0 0 0.01428571 0.02857143 0.04285714 0.05714286 0.07142857 0.08571429 0.1 0.11428571 0.12857143 0.14285714 0.15714286 0.17142857 0.18571429 0.2 0.21428571 0.22857143 0.24285714 0.25714286 0.27142857 0.28571429 0.3 0.31428571 0.32857143 0.34285714 0.35714286 0.37142857 0.38571429 0.4 0.41428571 0.42857143 0.44285714 0.45714286 0.47142857 0.48571429 0.5 0.51428571 0.52857143 0.54285714 0.55714286 0.57142857 0.58571429 0.6 0.61428571 0.62857143 0.64285714 0.65714286 0.67142857 0.68571429 0.7 0.71428571 0.72857143 0.74285714 0.75714286 0.77142857 0.78571429 0.8 0.81428571 0.82857143 0.84285714 0.85714286 0.87142857 0.88571429 0.9 0.91428571 0.92857143 0.94285714 0.95714286 0.97142857 0.98571429 1 1 1 1 1 1
  line L29 (6.957, -14.5353) -> (6.8123, -14.1977)
  arc A59 (7.2443, -13.0345) -> (6.8123, -14.1977) centre (7.6395, -13.8431) ccw
  arc A60 (7.2443, -13.0345) -> (7.7664, -12.7685) centre (-0.4607, 2.7328) ccw
  arc A61 (8.9614, -13.1027) -> (7.7664, -12.7685) centre (8.1883, -13.5635) ccw
  line L30 (8.9614, -13.1027) -> (9.1494, -13.4182)
  spline S30 degree 5 poles (9.1494, -13.4182) (9.1543, -13.4263) (9.1641, -13.4423) (9.1795, -13.466) (9.2012, -13.4968) (9.23, -13.5341) (9.2599, -13.5707) (9.2905, -13.6069) (9.3216, -13.6427) (9.3529, -13.6784) (9.3845, -13.7139) (9.4165, -13.7492) (9.449, -13.7841) (9.482, -13.8187) (9.5155, -13.8528) (9.5496, -13.8866) (9.5841, -13.92) (9.619, -13.9532) (9.6542, -13.9861) (9.6897, -14.0189) (9.7255, -14.0514) (9.7617, -14.0836) (9.7981, -14.1156) (9.8349, -14.1474) (9.872, -14.1788) (9.9095, -14.2101) (9.9472, -14.2411) (9.9853, -14.2718) (10.0236, -14.3024) (10.0622, -14.3327) (10.101, -14.3628) (10.1402, -14.3927) (10.1795, -14.4223) (10.2192, -14.4518) (10.2591, -14.481) (10.2993, -14.51) (10.3397, -14.5388) (10.3803, -14.5674) (10.4212, -14.5958) (10.4624, -14.6239) (10.5037, -14.6519) (10.5453, -14.6796) (10.5872, -14.7072) (10.6292, -14.7345) (10.6715, -14.7617) (10.714, -14.7886) (10.7567, -14.8153) (10.7996, -14.8419) (10.8428, -14.8682) (10.8861, -14.8943) (10.9297, -14.9203) (10.9734, -14.946) (11.0174, -14.9716) (11.0615, -14.9969) (11.1059, -15.0221) (11.1505, -15.047) (11.1952, -15.0718) (11.2402, -15.0963) (11.2853, -15.1207) (11.3306, -15.1449) (11.3761, -15.1689) (11.4218, -15.1927) (11.4677, -15.2163) (11.5137, -15.2397) (11.56, -15.263) (11.6064, -15.286) (11.653, -15.3088) (11.6997, -15.3315) (11.7467, -15.354) (11.7938, -15.3762) (11.841, -15.3983) (11.879, -15.4158) (11.9075, -15.4289) (11.9266, -15.4376) (11.9361, -15.4419) knots 0 0 0 0 0 0 0.01428571 0.02857143 0.04285714 0.05714286 0.07142857 0.08571429 0.1 0.11428571 0.12857143 0.14285714 0.15714286 0.17142857 0.18571429 0.2 0.21428571 0.22857143 0.24285714 0.25714286 0.27142857 0.28571429 0.3 0.31428571 0.32857143 0.34285714 0.35714286 0.37142857 0.38571429 0.4 0.41428571 0.42857143 0.44285714 0.45714286 0.47142857 0.48571429 0.5 0.51428571 0.52857143 0.54285714 0.55714286 0.57142857 0.58571429 0.6 0.61428571 0.62857143 0.64285714 0.65714286 0.67142857 0.68571429 0.7 0.71428571 0.72857143 0.74285714 0.75714286 0.77142857 0.78571429 0.8 0.81428571 0.82857143 0.84285714 0.85714286 0.87142857 0.88571429 0.9 0.91428571 0.92857143 0.94285714 0.95714286 0.97142857 0.98571429 1 1 1 1 1 1
  arc A62 (11.9361, -15.4419) -> (12.9936, -14.6736) centre (-0.4607, 2.7328) ccw
  spline S31 degree 5 poles (11.9301, -11.3979) (11.9363, -11.405) (11.9485, -11.4194) (11.9663, -11.4413) (11.9888, -11.4715) (12.0155, -11.5104) (12.041, -11.5501) (12.0659, -11.5904) (12.0904, -11.6311) (12.1147, -11.6719) (12.1387, -11.7129) (12.1623, -11.7542) (12.1855, -11.7959) (12.2082, -11.8379) (12.2303, -11.8804) (12.2519, -11.9233) (12.273, -11.9664) (12.2938, -12.0099) (12.3142, -12.0535) (12.3344, -12.0974) (12.3542, -12.1415) (12.3737, -12.1858) (12.3929, -12.2304) (12.4117, -12.2752) (12.4302, -12.3202) (12.4483, -12.3655) (12.4661, -12.411) (12.4836, -12.4567) (12.5008, -12.5025) (12.5178, -12.5486) (12.5344, -12.5949) (12.5507, -12.6413) (12.5668, -12.6879) (12.5825, -12.7347) (12.598, -12.7817) (12.6131, -12.8289) (12.628, -12.8762) (12.6426, -12.9237) (12.657, -12.9714) (12.6711, -13.0192) (12.6849, -13.0672) (12.6984, -13.1153) (12.7117, -13.1636) (12.7247, -13.2121) (12.7374, -13.2607) (12.7499, -13.3094) (12.7622, -13.3583) (12.7741, -13.4073) (12.7858, -13.4565) (12.7973, -13.5058) (12.8085, -13.5552) (12.8195, -13.6048) (12.8302, -13.6545) (12.8406, -13.7043) (12.8509, -13.7543) (12.8608, -13.8044) (12.8706, -13.8546) (12.88, -13.9049) (12.8893, -13.9554) (12.8983, -14.0059) (12.907, -14.0566) (12.9155, -14.1074) (12.9238, -14.1584) (12.9319, -14.2094) (12.9397, -14.2605) (12.9472, -14.3118) (12.9545, -14.3632) (12.9616, -14.4146) (12.9685, -14.4662) (12.9751, -14.5179) (12.9815, -14.5697) (12.9865, -14.6112) (12.9901, -14.6424) (12.9924, -14.6632) (12.9936, -14.6736) knots 0 0 0 0 0 0 0.01428571 0.02857143 0.04285714 0.05714286 0.07142857 0.08571429 0.1 0.11428571 0.12857143 0.14285714 0.15714286 0.17142857 0.18571429 0.2 0.21428571 0.22857143 0.24285714 0.25714286 0.27142857 0.28571429 0.3 0.31428571 0.32857143 0.34285714 0.35714286 0.37142857 0.38571429 0.4 0.41428571 0.42857143 0.44285714 0.45714286 0.47142857 0.48571429 0.5 0.51428571 0.52857143 0.54285714 0.55714286 0.57142857 0.58571429 0.6 0.61428571 0.62857143 0.64285714 0.65714286 0.67142857 0.68571429 0.7 0.71428571 0.72857143 0.74285714 0.75714286 0.77142857 0.78571429 0.8 0.81428571 0.82857143 0.84285714 0.85714286 0.87142857 0.88571429 0.9 0.91428571 0.92857143 0.94285714 0.95714286 0.97142857 0.98571429 1 1 1 1 1 1
  line L31 (11.9301, -11.3979) -> (11.6881, -11.1216)
  arc A63 (11.7396, -9.8818) -> (11.6881, -11.1216) centre (12.3653, -10.5287) ccw
  arc A64 (11.7396, -9.8818) -> (12.1539, -9.4675) centre (-0.4607, 2.7328) ccw
  arc A65 (13.3937, -9.4161) -> (12.1539, -9.4675) centre (12.8008, -10.0932) ccw
  line L32 (13.3937, -9.4161) -> (13.67, -9.658)
  spline S32 degree 5 poles (13.67, -9.658) (13.6771, -9.6642) (13.6914, -9.6764) (13.7134, -9.6942) (13.7435, -9.7167) (13.7824, -9.7434) (13.8222, -9.769) (13.8625, -9.7938) (13.9031, -9.8184) (13.944, -9.8426) (13.985, -9.8666) (14.0263, -9.8903) (14.0679, -9.9135) (14.11, -9.9361) (14.1525, -9.9582) (14.1953, -9.9798) (14.2385, -10.0009) (14.2819, -10.0217) (14.3256, -10.0422) (14.3695, -10.0623) (14.4136, -10.0822) (14.4579, -10.1017) (14.5025, -10.1208) (14.5473, -10.1397) (14.5923, -10.1581) (14.6376, -10.1763) (14.683, -10.1941) (14.7287, -10.2116) (14.7746, -10.2288) (14.8207, -10.2457) (14.8669, -10.2623) (14.9134, -10.2786) (14.96, -10.2947) (15.0068, -10.3104) (15.0538, -10.3259) (15.101, -10.3411) (15.1483, -10.356) (15.1958, -10.3706) (15.2435, -10.3849) (15.2913, -10.399) (15.3393, -10.4128) (15.3874, -10.4263) (15.4357, -10.4396) (15.4841, -10.4526) (15.5327, -10.4654) (15.5815, -10.4779) (15.6303, -10.4901) (15.6794, -10.5021) (15.7285, -10.5138) (15.7778, -10.5252) (15.8273, -10.5364) (15.8768, -10.5474) (15.9265, -10.5581) (15.9764, -10.5686) (16.0263, -10.5788) (16.0764, -10.5888) (16.1266, -10.5985) (16.177, -10.608) (16.2274, -10.6172) (16.278, -10.6262) (16.3287, -10.635) (16.3795, -10.6435) (16.4304, -10.6517) (16.4815, -10.6598) (16.5326, -10.6676) (16.5839, -10.6752) (16.6352, -10.6825) (16.6867, -10.6896) (16.7383, -10.6964) (16.79, -10.7031) (16.8418, -10.7095) (16.8833, -10.7144) (16.9145, -10.718) (16.9353, -10.7203) (16.9457, -10.7215) knots 0 0 0 0 0 0 0.01428571 0.02857143 0.04285714 0.05714286 0.07142857 0.08571429 0.1 0.11428571 0.12857143 0.14285714 0.15714286 0.17142857 0.18571429 0.2 0.21428571 0.22857143 0.24285714 0.25714286 0.27142857 0.28571429 0.3 0.31428571 0.32857143 0.34285714 0.35714286 0.37142857 0.38571429 0.4 0.41428571 0.42857143 0.44285714 0.45714286 0.47142857 0.48571429 0.5 0.51428571 0.52857143 0.54285714 0.55714286 0.57142857 0.58571429 0.6 0.61428571 0.62857143 0.64285714 0.65714286 0.67142857 0.68571429 0.7 0.71428571 0.72857143 0.74285714 0.75714286 0.77142857 0.78571429 0.8 0.81428571 0.82857143 0.84285714 0.85714286 0.87142857 0.88571429 0.9 0.91428571 0.92857143 0.94285714 0.95714286 0.97142857 0.98571429 1 1 1 1 1 1
  arc A66 (16.9457, -10.7215) -> (17.7139, -9.6641) centre (-0.4607, 2.7328) ccw